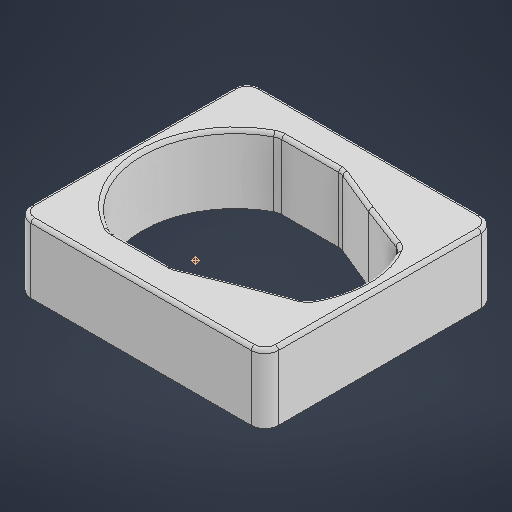
# Autodesk Inventor part: PipetteProfile
Saved by Autodesk Inventor 2025.1 (Build 291241000, 241)
## iProperties
Created: 2024-10-27
Part Number: PipetteProfile
Material: Generic
Document SubType Name: Modeling
Designer: 13156
Density: 1 g/cm^3
Appearance: Default
Author: 13156
## iProperties of the stored document PipetteProfile_3DPrint.ipt
Created: 2024-10-27
Part Number: PipetteProfile_3DPrint
Material: Generic
Document SubType Name: Modeling
Designer: jerem
Density: 1 g/cm^3
Appearance: Default
Author: jerem
Autodesk Inventor part; units mm, degrees
ref_plane "YZ Plane" through (0, 0, 0) normal (1, 0, 0) x (0, 1, 0)
ref_plane "XZ Plane" through (0, 0, 0) normal (0, 1, 0) x (-1, 0, 0)
ref_plane "XY Plane" through (0, 0, 0) normal (0, 0, 1) x (1, 0, 0)
sketch "Sketch6" plane through (0, 0, 0) normal (0, 1, 0) x (-1, 0, 0)
  arc A0 (0, -12.3) -> (0, 12.3) centre (-5.974, 0) ccw
  line L0 (0, -23.7314) -> (0, 23.4378) projected
  line L1 (0, 12.3) -> (-9.2, 12.3)
  line L2 (0, -12.3) -> (-9.2, -12.3)
  line L3 (-9.2, 12.3) -> (-16, 9.5)
  line L4 (-9.2, -12.3) -> (-16, -9.5)
  line L5 (-16, 9.5) -> (-23.1, 6.8)
  line L6 (-16, -9.5) -> (-23.1, -6.8)
  arc A1 (-23.1, 6.8) -> (-23.1, -6.8) centre (-12.54, 0) ccw
  line L7 (9.3004, 16.6993) -> (-26.9762, 16.6993)
  line L8 (-26.9762, 16.6993) -> (-26.9762, -16.993)
  line L9 (-26.9762, -16.993) -> (9.3004, -16.993)
  line L10 (9.3004, -16.993) -> (9.3004, 16.6993)
  point P0 (0, 0)
  point P1 (7.7, 0)
  point P2 (-25.1, 0)
  dimension "d4" = 0
  dimension "d6" = 0
  dimension "d7" = 7.7
  dimension "d8" = 9.2
  dimension "d9" = 9.2
  dimension "d10" = 2.8
  dimension "d11" = 2.8
  dimension "d12" = 6.8
  dimension "d13" = 6.8
  dimension "d15" = 24.6
  dimension "d16" = 7.1
  dimension "d17" = 7.1
  dimension "d18" = 2.7
  dimension "d19" = 2.7
  dimension "d20" = 2
  constraints: 20 end point, 6 point on circle, 3 horizontal, 2 centre point, 2 parallel, 1 perpendicular
  measures "d4" vertical distance of point (7.7, 0) point (0, 0)
  measures "d6" distance from line of L0 L1.start
  measures "d7" distance from line of L0 point (7.7, 0)
  measures "d8" distance of L1.start L1.end
  measures "d9" distance of L2.start L2.end
  measures "d10" vertical distance of L3.end L1.end
  measures "d11" vertical distance of L4.end L2.end
  measures "d12" horizontal distance of L4.end L2.end
  measures "d13" horizontal distance of L3.end L1.end
  measures "d15" distance of L2.start L1.start
  measures "d16" horizontal distance of L5.end L3.end
  measures "d17" horizontal distance of L6.end L4.end
  measures "d18" vertical distance of L4.end L6.end
  measures "d19" vertical distance of L3.end L5.end
  measures "d20" horizontal distance of L6.end point (-25.1, 0)
extrude "Extrusion1" add sketch "Sketch6" along normal blind 10 contours A0 L0 L7 L10 L9 | L0 L9 L8 L7 L1 L3 L5 A1 L6 L4 L2
fillet "Fillet1" radius 2 8 edges at (0, 5, -12.3) (9.2, 5, -12.3) (16, 5, -9.5) (23.1, 5, -6.8) (23.1, 5, 6.8) (16, 5, 9.5) (9.2, 5, 12.3) (0, 5, 12.3)
fillet "Fillet2" radius 2 4 edges at (26.9762, 5, -16.993) (-9.3004, 5, -16.993) (-9.3004, 5, 16.6993) (26.9762, 5, 16.6993)
fillet "Fillet3" radius 0.5 8 edges at (26.3904, 10, -16.4072) (8.8379, 10, -16.993) (-8.7146, 10, -16.4072) (-9.3004, 10, -0.1468) (-8.7146, 10, 16.1135) (8.8379, 10, 16.6993) (26.3904, 10, 16.1135) (26.9762, 10, -0.1468)
fillet "Fillet4" radius 0.5 14 edges at (-0.006, 10, -12.2403) (4.6418, 10, -12.3) (9.1925, 10, -12.262) (12.7829, 10, -10.8247) (23.0498, 10, -6.6911) (19.2278, 10, -8.2725) (25.1, 10, 0) (23.0498, 10, 6.6911) (19.2278, 10, 8.2725) (9.1925, 10, 12.262) (12.7829, 10, 10.8247) (4.6418, 10, 12.3) (-0.006, 10, 12.2403) (-7.7, 10, 0)
body "Solid1"
